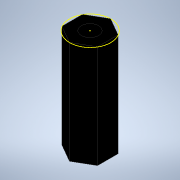
# Autodesk Inventor part: testtt
Saved by Autodesk Inventor 2021 (Build 250183000, 183)
## iProperties
Created: 2025-02-01
Part Number: testtt
Material: Generic
Document SubType Name: Modeling
Designer: 22liatho
Density: 1 g/cm^3
Appearance: Default
Author: 22liatho
Autodesk Inventor part; units mm, degrees
ref_plane "YZ Plane" through (0, 0, 0) normal (1, 0, 0) x (0, 1, 0)
ref_plane "XZ Plane" through (0, 0, 0) normal (0, 1, 0) x (-1, 0, 0)
ref_plane "XY Plane" through (0, 0, 0) normal (0, 0, 1) x (1, 0, 0)
sketch "Sketch1" plane through (0, 0, 0) normal (0, 1, 0) x (-1, 0, 0)
  circle A0 centre (0, 0) radius 1.25
  line L0 (0, -3) -> (-2.5981, -1.5)
  line L1 (-2.5981, -1.5) -> (-2.5981, 1.5)
  line L2 (-2.5981, 1.5) -> (0, 3)
  line L3 (0, 3) -> (2.5981, 1.5)
  line L4 (2.5981, 1.5) -> (2.5981, -1.5)
  line L5 (2.5981, -1.5) -> (0, -3)
  circle A1 centre (0, 0) radius 3
  dimension "d0" = 2.5
  dimension "d12" = 6
  constraints: 12 end point, 3 coincident, 1 centre point, 1 vertical, 1 vertical alignment, 15 other
  measures "d0" diameter of A0
  measures "d12" distance of L2.end L0.start
extrude "Extrusion1" add sketch "Sketch1" along normal blind 15 contours L0 L1 L2 L3 L4 L5
sketch "Sketch2" plane through (0, 0, 0) normal (1, 0, 0) x (0, 1, 0)
  line L0 (15.9, -0.8603) -> (15.675, -1.25)
  line L1 (15.675, -1.25) -> (15.45, -0.8603)
  line L2 (15.45, -0.8603) -> (15.9, -0.8603)
  line L3 (15, 1.25) -> (15, -1.25) projected
  line L4 (15, 1.25) -> (15, -1.25) projected
  line L5 (0, 1.25) -> (0, -1.25) projected
  line L6 (15, 1.5) -> (15, -1.5) projected
  line L7 (15, 0) -> (16, 0)
  point P0 (0, 0)
  dimension "d4" = 60
  dimension "d5" = 60
  dimension "d6" = 0.45
  dimension "d7" = 1
  dimension "d8" = 1.25
  dimension "d11" = 0.45
  constraints: 8 end point, 2 horizontal, 1 midpoint
  measures "d4" angle of L2 L1
  measures "d5" angle of L0 L2
  measures "d6" distance of L1.end L0.start
  measures "d7" distance of L7.start L7.end
  measures "d8" distance from line of L7 L0.end
  measures "d11" distance from line of L6 L1.end
sketch "Sketch3" plane through (0, 15, 0) normal (0, 1, 0) x (1, 0, 0)
  circle A0 centre (0, 0) radius 3 projected
equation "\"d6\" = d11"
body "Solid1"
